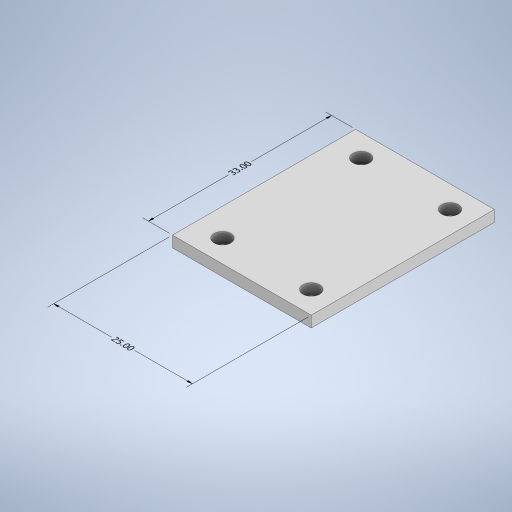
# Autodesk Inventor part: CamBracket
Saved by Autodesk Inventor 2024 (Build 280153000, 153)
## iProperties
Created: 2023-05-15
Part Number: CamBracket
Material: Generic
Document SubType Name: Modeling
Designer: User
Density: 1 g/cm^3
Appearance: Default
Author: User
Autodesk Inventor part; units mm, degrees
ref_plane "YZ Plane" through (0, 0, 0) normal (1, 0, 0) x (0, 1, 0)
ref_plane "XZ Plane" through (0, 0, 0) normal (0, 1, 0) x (-1, 0, 0)
ref_plane "XY Plane" through (0, 0, 0) normal (0, 0, 1) x (1, 0, 0)
sketch "Sketch3" plane through (0, 0, 0) normal (0, 1, 0) x (-1, 0, 0)
  line L0 (0, 0) -> (25, 0)
  line L1 (25, 0) -> (25, -33)
  line L2 (25, -33) -> (0, -33)
  line L3 (0, -33) -> (0, 0)
  dimension "d6" = 25
  dimension "d7" = 33
  constraints: 8 end point, 2 parallel, 1 horizontal, 1 perpendicular
  measures "d6" distance of L1.end L2.end
  measures "d7" distance of L0.end L1.end
extrude "Extrusion2" add sketch "Sketch3" along normal blind 2
sketch "Sketch4" plane through (0, 2, 0) normal (0, 1, 0) x (1, 0, 0)
  circle A0 centre (-4, 4) radius 1.5
  line L0 (0, 0) -> (0, 33) projected
  line L1 (-25, 0) -> (0, 0) projected
  circle A1 centre (-4, 29) radius 1.5
  line L2 (0, 33) -> (-25, 33) projected
  circle A2 centre (-20, 4) radius 1.5
  line L3 (-25, 33) -> (-25, 0) projected
  circle A3 centre (-20, 29) radius 1.5
  dimension "d16" = 3
  dimension "d17" = 4
  dimension "d18" = 4
  dimension "d19" = 3
  dimension "d20" = 4
  dimension "d21" = 4
  dimension "d22" = 3
  dimension "d23" = 16
  dimension "d24" = 4
  dimension "d25" = 5
  dimension "d26" = 3
  dimension "d27" = 4
  dimension "d28" = 16
  dimension "d29" = 25
  constraints: 4 centre point
  measures "d16" diameter of A0
  measures "d17" distance from line of L0 A0.centre
  measures "d18" distance from line of L1 A0.centre
  measures "d19" diameter of A1
  measures "d20" distance from line of L0 A1.centre
  measures "d21" distance from line of L2 A1.centre
  measures "d22" diameter of A2
  measures "d23" distance of A0.centre A2.centre
  measures "d24" distance from line of L1 A2.centre
  measures "d25" distance from line of L3 A2.centre
  measures "d26" diameter of A3
  measures "d27" distance from line of L2 A3.centre
  measures "d28" distance of A1.centre A3.centre
  measures "d29" distance of A1.centre A0.centre
extrude "Extrusion3" cut sketch "Sketch4" against normal blind 2 contours A0 | A1 | A2 | A3
body "Solid2"
